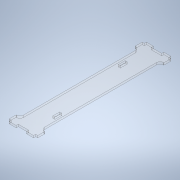
# Autodesk Inventor part: camRiser
Saved by Autodesk Inventor 2020 (Build 240168000, 168)
## iProperties
Created: 2019-08-06
Part Number: camRiser
Material: Polycarbonate, Clear
Document SubType Name: Modeling
Designer: n10208577
Density: 1.2 g/cm^3
Appearance: Polycarbonate - Clear
Author: n10208577
Autodesk Inventor part; units mm, degrees
ref_plane "YZ Plane" through (0, 0, 0) normal (1, 0, 0) x (0, 1, 0)
ref_plane "XZ Plane" through (0, 0, 0) normal (0, 1, 0) x (-1, 0, 0)
ref_plane "XY Plane" through (0, 0, 0) normal (0, 0, 1) x (1, 0, 0)
sketch "Sketch1" plane through (0, 0, 0) normal (0, 1, 0) x (-1, 0, 0)
  line L0 (11.4156, -82.4999) -> (11.4156, 77.5001)
  arc A0 (6.4156, -87.4999) -> (11.4156, -82.4999) centre (6.4156, -82.4999) ccw
  arc A1 (11.4156, 77.5001) -> (6.4156, 82.5001) centre (6.4156, 77.5001) ccw
  line L1 (41.4156, 77.5001) -> (41.4156, -82.4999)
  line L2 (33.9156, -97.4999) -> (33.9156, -100.4999)
  line L3 (33.9156, -100.4999) -> (43.9156, -100.4999)
  line L4 (43.9156, -100.4999) -> (43.9156, -97.4999)
  line L5 (18.9156, -97.4999) -> (18.9156, -100.4999)
  line L6 (18.9156, -100.4999) -> (8.9156, -100.4999)
  line L7 (8.9156, -100.4999) -> (8.9156, -97.4999)
  line L8 (18.9156, -97.4999) -> (33.9156, -97.4999)
  line L9 (8.9156, -97.4999) -> (5.9156, -97.4999)
  line L10 (5.9156, -97.4999) -> (5.9156, -87.4999)
  line L11 (5.9156, -87.4999) -> (6.4156, -87.4999)
  line L12 (43.9156, -97.4999) -> (46.9156, -97.4999)
  line L13 (46.9156, -97.4999) -> (46.9156, -87.4999)
  line L14 (46.9156, -87.4999) -> (46.4156, -87.4999)
  arc A2 (41.4156, -82.4999) -> (46.4156, -87.4999) centre (46.4156, -82.4999) ccw
  line L15 (18.9156, 92.5001) -> (18.9156, 95.5001)
  line L16 (18.9156, 95.5001) -> (8.9156, 95.5001)
  line L17 (8.9156, 95.5001) -> (8.9156, 92.5001)
  line L18 (33.9156, 92.5001) -> (33.9156, 95.5001)
  line L19 (33.9156, 95.5001) -> (43.9156, 95.5001)
  line L20 (43.9156, 95.5001) -> (43.9156, 92.5001)
  line L21 (33.9156, 92.5001) -> (18.9156, 92.5001)
  line L22 (43.9156, 92.5001) -> (46.9156, 92.5001)
  line L23 (46.9156, 92.5001) -> (46.9156, 82.5001)
  line L24 (46.9156, 82.5001) -> (46.4156, 82.5001)
  arc A3 (46.4156, 82.5001) -> (41.4156, 77.5001) centre (46.4156, 77.5001) ccw
  line L25 (8.9156, 92.5001) -> (5.9156, 92.5001)
  line L26 (5.9156, 92.5001) -> (5.9156, 82.5001)
  line L27 (5.9156, 82.5001) -> (6.4156, 82.5001)
  line L28 (33.4156, -52.6499) -> (33.4156, -62.3499)
  line L29 (33.4156, -62.3499) -> (36.2156, -62.3499)
  line L30 (36.2156, -57.4999) -> (36.2156, -52.6499)
  line L31 (36.2156, -52.6499) -> (33.4156, -52.6499)
  line L32 (36.2156, -57.4999) -> (36.2156, -62.3499)
  line L33 (16.6156, 47.6501) -> (16.6156, 57.3501)
  line L34 (16.6156, 57.3501) -> (19.4156, 57.3501)
  line L35 (19.4156, 52.5001) -> (19.4156, 47.6501)
  line L36 (19.4156, 47.6501) -> (16.6156, 47.6501)
  line L37 (19.4156, 52.5001) -> (19.4156, 57.3501)
  constraints: 76 end point, 8 point on circle, 4 centre point
extrude "Extrusion1" add sketch "Sketch1" along normal blind 3
body "Solid1"
